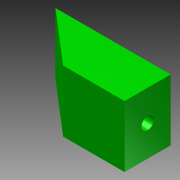
# Autodesk Inventor part: BatteryLatch-Latch
Saved by Autodesk Inventor 2012 (Build 160160000, 160)
## iProperties
Created: 2013-10-13
Part Number: BatteryLatch-Latch
Material: Default
Document SubType Name: Modeling
Designer: joe_000
Density: 1 g/cm^3
plungerWidth: 0.375 in
plungerLength: 0.500 in
plungerHeight: 0.500 in
latchLength: 0.438 in
plungerTolerance: 0.063 in
Author: joe_000
Autodesk Inventor part; units mm, degrees
ref_plane "YZ Plane" through (0, 0, 0) normal (1, 0, 0) x (0, 1, 0)
ref_plane "XZ Plane" through (0, 0, 0) normal (0, 1, 0) x (-1, 0, 0)
ref_plane "XY Plane" through (0, 0, 0) normal (0, 0, 1) x (1, 0, 0)
sketch "Sketch1" plane through (0, 0, 0) normal (0, 1, 0) x (-1, 0, 0)
  line L0 (0, 0) -> (-11.1125, 9.525)
  line L1 (-11.1125, 9.525) -> (-23.8125, 9.525)
  line L2 (-23.8125, 9.525) -> (-23.8125, 0)
  line L3 (-23.8125, 0) -> (0, 0)
  dimension "plungerWidth" = 9.525
  dimension "plungerLength" = 12.7
  dimension "latchLength" = 11.1125
  constraints: 8 end point, 2 perpendicular, 1 horizontal
  measures "plungerWidth" distance of L1.end L2.end
  measures "plungerLength" distance of L0.end L1.end
  measures "latchLength" horizontal distance of L0.start L0.end
extrude "Extrusion1" add sketch "Sketch1" against normal blind 12.7
sketch "Sketch2" plane through (23.8125, 0, 9.525) normal (1, 0, 0) x (0, 0, -1)
  circle A0 centre (4.7625, -6.35) radius 1.27
  line L0 (0, 0) -> (9.525, 0) projected
  line L1 (0, 0) -> (0, -12.7) projected
  dimension "screwDiameter" = 2.54
  dimension "d8" = 6.35
  dimension "d9" = 4.7625
  constraints: 1 centre point
  measures "screwDiameter" diameter of A0
  measures "d8" distance from line of L0 A0.centre
  measures "d9" distance from line of L1 A0.centre
extrude "Extrusion2" cut sketch "Sketch2" against normal blind 12.7
equation "\"d8\" = 0.5 * plungerHeight"
equation "\"d9\" = 0.5 * plungerWidth"
equation "\"screwDepth\" = plungerLength"
equation "\"plungerTolerance\" = 1.5875"
equation "\"plungerHeight\" = 12.7"
body "Solid1"
